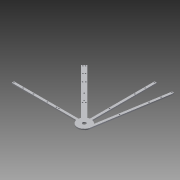
# Autodesk Inventor part: Bearing Mount v1
Saved by Autodesk Inventor 2013 (Build 170138000, 138)
## iProperties
Created: 2013-01-15
Part Number: Bearing Mount v1
Material: Aluminum 6061
Document SubType Name: Modeling
Designer: actoennies
Mass: 447.684 g
Surface Area: 757.559 cm^2
Volume: 165.197 cm^3
Density: 2.71 g/cm^3
Author: actoennies
Autodesk Inventor part; units mm, degrees
ref_plane "YZ Plane" through (0, 0, 0) normal (1, 0, 0) x (0, 1, 0)
ref_plane "XZ Plane" through (0, 0, 0) normal (0, 1, 0) x (-1, 0, 0)
ref_plane "XY Plane" through (0, 0, 0) normal (0, 0, 1) x (1, 0, 0)
sketch "Sketch1" plane through (0, 0, 0) normal (0, 1, 0) x (-1, 0, 0)
  line L0 (269.2628, -287.2233) -> (16.4197, -34.3803)
  circle A0 centre (270.2276, -277.5195) radius 3.3782
  line L1 (287.2233, -269.2628) -> (34.3803, -16.4197)
  line L2 (6.35, -37.5671) -> (6.35, -393.6488)
  line L3 (-6.35, -37.5671) -> (-6.35, -393.7)
  line L4 (-90.8271, -393.7) -> (-29.6915, -23.8752)
  line L5 (-101.6, -381) -> (-37.5898, 6.214)
  circle A1 centre (0, -387.35) radius 3.3782
  line L6 (37.5671, 6.35) -> (393.7, 6.35)
  line L7 (37.5671, -6.35) -> (393.6488, -6.35)
  circle A2 centre (387.35, 0) radius 3.3782
  circle A3 centre (-95.25, -387.35) radius 3.3782
  circle A4 centre (277.5195, -270.2276) radius 3.3782
  line L8 (-101.6, -381) -> (-101.6, -393.7)
  line L9 (393.7, 0) -> (393.7, 6.35)
  arc A5 (6.35, -37.5671) -> (16.4197, -34.3803) centre (0, 0) ccw
  arc A6 (34.3803, -16.4197) -> (37.5671, -6.35) centre (0, 0) ccw
  line L10 (38.1, 0) -> (38.1, 12.8556) construction
  arc A7 (37.5671, 6.35) -> (-37.5898, 6.214) centre (0, 0) ccw
  circle A8 centre (0, 0) radius 38.1 construction
  arc A9 (-6.214, 37.5898) -> (-37.5898, 6.214) centre (0, 0) ccw
  arc A10 (-29.6915, -23.8752) -> (-6.35, -37.5671) centre (0, 0) ccw
  line L11 (146.05, 0) -> (146.05, 6.35)
  line L12 (133.35, 0) -> (133.35, 6.35)
  line L13 (273.05, 6.35) -> (273.05, 0)
  line L14 (285.75, 6.35) -> (285.75, 0)
  circle A11 centre (103.1708, -94.1906) radius 3.3782
  circle A12 centre (94.1906, -103.1708) radius 3.3782
  arc A13 (393.6488, -6.35) -> (393.7, 0) centre (0, 0) ccw
  circle A14 centre (279.4, 0) radius 3.3782
  circle A15 centre (139.7, 0) radius 3.3782
  arc A16 (0, -393.7) -> (6.35, -393.6488) centre (0, 0) ccw
  arc A17 (269.2628, -287.2233) -> (287.2233, -269.2628) centre (0, 0) ccw
  circle A18 centre (202.0047, -193.0245) radius 3.3782
  circle A19 centre (193.0245, -202.0047) radius 3.3782
  circle A20 centre (0, -279.4) radius 3.3782
  line L15 (-101.6, -393.7) -> (-90.8271, -393.7)
  line L16 (-6.35, -393.7) -> (0, -393.7)
  circle A21 centre (0, -139.7) radius 3.3782
  circle A22 centre (0, 0) radius 14.2875
  circle A23 centre (-55.2746, -139.7) radius 3.3782
  circle A24 centre (-78.3684, -279.4) radius 3.3782
  line L17 (0, -285.75) -> (-6.35, -285.75)
  line L18 (-6.35, -273.05) -> (0, -273.05)
  circle A25 centre (0, -336.55) radius 3.3782
  circle A26 centre (-87.8158, -336.55) radius 3.3782
  circle A27 centre (241.5985, -234.3065) radius 3.3782
  circle A28 centre (234.3065, -241.5985) radius 3.3782
  circle A29 centre (336.55, 0) radius 3.3782
  dimension "d0" = 12.7
  dimension "d1" = 101.6
  dimension "d2" = 12.7
  dimension "d3" = 12.7
  dimension "d4" = 38.1
  dimension "d5" = 38.1
  dimension "d6" = 38.1
  dimension "d7" = 6.35
  dimension "d8" = 6.35
  dimension "d9" = 6.35
  dimension "d10" = 12.7
  dimension "d11" = 12.7
  dimension "d12" = 95.25
  dimension "d14" = 6.7564
  dimension "d15" = 6.7564
  dimension "d16" = 6.7564
  dimension "d17" = 6.35
  dimension "d18" = 6.7564
  dimension "d19" = 6.35
  dimension "d20" = 6.35
  dimension "d21" = 6.7564
  dimension "d22" = 6.7564
  dimension "d23" = 6.7564
  dimension "d25" = 6.35
  dimension "d26" = 6.7564
  dimension "d28" = 28.575
  dimension "d30" = 6.7564
  dimension "d32" = 6.7564
  dimension "d36" = 38.1
  dimension "d37" = 25.4
  dimension "d38" = 6.35
  dimension "d39" = 139.7
  dimension "d40" = 55.2746
  dimension "d41" = 139.7
  dimension "d42" = 6.35
  dimension "d43" = 6.35
  dimension "d44" = 7.3006
  dimension "d45" = 277.5195
  dimension "d46" = 270.2276
  dimension "d47" = 7.2919
  dimension "d48" = 7.2919
  dimension "d49" = 393.7
  dimension "d50" = 393.7
  dimension "d51" = 6.35
  dimension "d52" = 12.7
  dimension "d53" = 6.7564
  dimension "d54" = 6.35
  dimension "d55" = 6.7564
  dimension "d56" = 6.7564
  dimension "d57" = 393.7
  dimension "d58" = 6.35
  dimension "d60" = 6.7564
  dimension "d61" = 6.35
  dimension "d62" = 6.7564
  dimension "d63" = 6.7564
  dimension "d64" = 6.7564
  dimension "d65" = 6.7564
  dimension "d66" = 50.8
  dimension "d67" = 50.8
  dimension "d68" = 50.8
  dimension "d71" = 7.5438
  dimension "d72" = 7.5438
  dimension "d73" = 7.5438
  dimension "d74" = 7.5438
  constraints: 38 end point, 30 centre point, 18 point on circle, 6 point on line, 5 parallel, 5 perpendicular, 2 coincident, 2 tangent
  measures "d0" distance between parallel lines of L4 L5
  measures "d1" distance of L8.end L16.end
  measures "d2" distance from line of L0 A17.centre
  measures "d3" distance from line of A17.centre L1
  measures "d4" radius of A9
  measures "d5" radius of A10
  measures "d6" radius of A5
  measures "d7" distance from line of L3 A17.centre
  measures "d8" distance from line of A17.centre L2
  measures "d9" distance from line of L6 A17.centre
  measures "d10" distance between parallel lines of L11 L12
  measures "d11" distance between parallel lines of L13 L14
  measures "d12" distance from line of L12 L10.start
  measures "d14" diameter of A11
  measures "d15" diameter of A12
  measures "d16" diameter of A14
  measures "d17" distance from line of L6 A14.centre
  measures "d18" diameter of A15
  measures "d19" distance from line of L6 A15.centre
  measures "d20" distance from line of L11 A15.centre
  measures "d21" diameter of A18
  measures "d22" diameter of A19
  measures "d23" diameter of A20
  measures "d25" distance from line of L3 A20.centre
  measures "d26" diameter of A21
  measures "d28" diameter of A22
  measures "d30" diameter of A23
  measures "d32" diameter of A24
  measures "d36" radius of A6
  measures "d37" distance from line of point (0, 0) L4
  measures "d38" distance from line of point (0, 0) L3
  measures "d39" distance of point (0, 0) A21.centre
  measures "d40" distance of A21.centre A23.centre
  measures "d41" vertical distance of A23.centre point (0, 0)
  measures "d42" distance from line of L2 A1.centre
  measures "d43" distance from line of L4 A24.centre
  measures "d44" distance from line of L5 A3.centre
  measures "d45" vertical distance of A17.centre A0.centre
  measures "d46" horizontal distance of point (0, 0) A0.centre
  measures "d47" horizontal distance of A0.centre A4.centre
  measures "d48" horizontal distance of A0.centre A4.centre
  measures "d49" radius of A17
  measures "d50" radius of A13
  measures "d51" distance of L9.start L6.end
  measures "d52" distance between parallel lines of L7 L6
  measures "d53" diameter of A2
  measures "d54" distance from line of L7 A2.centre
  measures "d55" diameter of A4
  measures "d56" diameter of A0
  measures "d57" radius of A16
  measures "d58" distance of L3.end L16.end
  measures "d60" diameter of A25
  measures "d61" distance of L16.end A1.centre
  measures "d62" diameter of A26
  measures "d63" diameter of A27
  measures "d64" diameter of A28
  measures "d65" diameter of A29
  measures "d66" distance of A2.centre A29.centre
  measures "d67" distance of A4.centre A27.centre
  measures "d68" distance of A0.centre A28.centre
  measures "d71" distance from line of L1 A27.centre
  measures "d72" distance from line of L0 A28.centre
  measures "d73" distance from line of L0 A0.centre
  measures "d74" distance from line of L1 A4.centre
extrude "Extrusion2" add sketch "Sketch1" along normal blind 6.35
sketch "Sketch6" plane through (0, 6.35, 0) normal (0, 1, 0) x (1, 0, 0)
  line L0 (-16.4197, 34.3803) -> (-269.2628, 287.2233) projected
  line L1 (-287.2233, 269.2628) -> (-34.3803, 16.4197) projected
  line L2 (-393.7, -6.35) -> (-37.5671, -6.35) projected
  line L3 (101.6, 381) -> (101.6, 393.7) projected
  arc A0 (0, 393.7) -> (-6.35, 393.6488) centre (0, 0) ccw projected
  line L4 (0, 0) -> (-287.2233, 287.2233) construction
  circle A1 centre (0, 0) radius 14.2875 projected
  line L5 (-37.5671, 6.35) -> (-393.6488, 6.35) projected
  line L6 (6.35, 37.5671) -> (6.35, 393.7) projected
  circle A2 centre (-107.7631, 107.7631) radius 3.3782
  circle A3 centre (-143.6841, 143.6841) radius 3.3782
  line L7 (-146.05, 464.3998) -> (-146.05, -90.5947) construction
  circle A4 centre (-203.2, 0) radius 3.3782
  circle A5 centre (-152.4, 0) radius 3.3782
  line L8 (-146.05, -6.35) -> (-146.05, 6.35)
  line L9 (-209.55, 6.35) -> (-209.55, -6.35)
  line L10 (-139.194, 157.1545) -> (-157.1545, 139.194)
  line L11 (-112.2532, 94.2927) -> (-94.2927, 112.2532)
  line L12 (-209.55, 6.35) -> (-157.1545, 139.194)
  line L13 (-112.2532, 94.2927) -> (-146.05, 6.35)
  line L14 (-183.3522, 72.772) -> (-129.1516, 50.3213)
  dimension "d115" = 6.7564
  dimension "d117" = 6.7564
  dimension "d118" = 247.65
  dimension "d122" = 152.4
  dimension "d123" = 203.2
  dimension "d124" = 6.7564
  dimension "d126" = 152.4
  dimension "d127" = 203.2
  dimension "d129" = 6.35
  dimension "d130" = 6.35
  dimension "d131" = 6.35
  dimension "d132" = 6.35
  constraints: 18 end point, 10 point on line, 4 centre point, 3 perpendicular, 2 midpoint, 2 parallel, 1 collinear
  measures "d115" diameter of A2
  measures "d117" diameter of A3
  measures "d118" distance between parallel lines of L7 L3
  measures "d122" distance of L4.start A2.centre
  measures "d123" distance of L4.start A3.centre
  measures "d124" diameter of A4
  measures "d126" distance of A1.centre A5.centre
  measures "d127" distance of L4.start A4.centre
  measures "d129" distance from line of L9 A4.centre
  measures "d130" distance from line of L8 A5.centre
  measures "d131" distance from line of L10 A3.centre
  measures "d132" distance from line of A2.centre L11
extrude "Extrusion8" cut sketch "Sketch6" against normal blind 25.4 contours A2 | A3 | A4 | A5
sketch "Sketch8" plane through (0, 6.35, 0) normal (0, 1, 0) x (1, 0, 0)
  circle A0 centre (0, 0) radius 14.2875 projected
  arc A1 (0, 393.7) -> (-6.35, 393.6488) centre (0, 0) ccw projected
  circle A2 centre (0, 0) radius 9.5
  dimension "d135" = 19
  constraints: 1 centre point, 1 coincident
  measures "d135" diameter of A2
extrude "Extrusion9" add sketch "Sketch8" against normal blind 6.35
equation "\"d71\" = d74"
equation "\"d72\" = d73"
body "Solid2"
